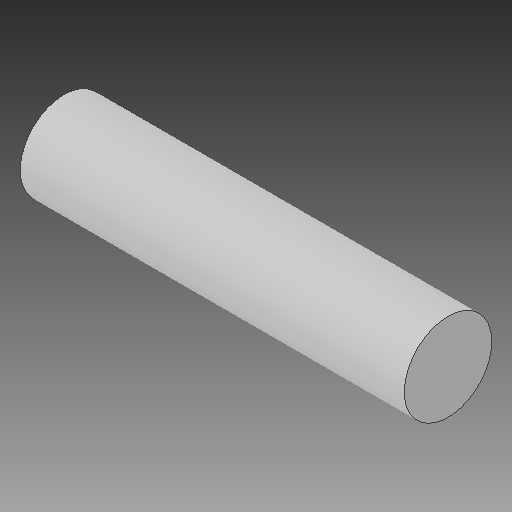
# Autodesk Inventor part: Shaft_8mm
Saved by Autodesk Inventor 2019.3 (Build 233278000, 278)
## iProperties
Created: 2020-08-24
Part Number: Shaft_8mm
Material: Generisch
Document SubType Name: Modeling
Designer: Nicolas Frick
Density: 1 g/cm^3
Appearance: Vorgabe
Mass: 1.75051 g
Surface Area: 9.77476 cm^2
Volume: 1.75051 cm^3
Author: Nicolas Frick
Autodesk Inventor part; units mm, degrees
ref_plane "YZ Plane" through (0, 0, 0) normal (1, 0, 0) x (0, 1, 0)
ref_plane "XZ Plane" through (0, 0, 0) normal (0, 1, 0) x (-1, 0, 0)
ref_plane "XY Plane" through (0, 0, 0) normal (0, 0, 1) x (1, 0, 0)
sketch "Skizze2" plane through (0, 0, 0) normal (0, 0, 1) x (1, 0, 0)
  line L0 (0, 7.8) -> (0, -7.8) construction
  line L1 (40, -7.8) -> (40, 7.8) construction
  line L2 (40, 0) -> (40, 3.9902) construction
  line L3 (5, 4.2) -> (5, -4.2) construction
  line L4 (35, -4.2) -> (35, 4.2) construction
  line L5 (35, 3.9902) -> (34.1, 3.9902) construction
  line L6 (34.1, 2.9902) -> (35, 2.9902) construction
  line L7 (40, 3.9902) -> (35, 3.9902) construction
  line L8 (0, 0) -> (31.65, 0) construction
  line L9 (31.65, 0) -> (31.65, 3.99) construction
  line L10 (31.65, 3.99) -> (0, 3.99) construction
  line L11 (0, 3.99) -> (0, 0) construction
  line L12 (0, 3.99) -> (35, 3.99)
  line L13 (35, 3.99) -> (35, 0)
  line L14 (35, 0) -> (0, 0)
  line L15 (0, 0) -> (0, 3.99)
  constraints: 24 end point, 5 parallel, 3 horizontal, 2 perpendicular, 2 point on line, 1 midpoint
revolve "Umdrehung2" add sketch "Skizze2" angle 360 about axis through (0, 0, 0) along (1, 0, 0)
